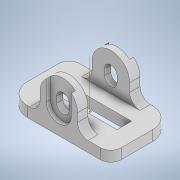
# Autodesk Inventor part: 15-1
Saved by Autodesk Inventor 2022 (Build 260153000, 153)
## iProperties
Created: 2021-09-25
Part Number: 15-1
Material: 일반
Document SubType Name: Modeling
Designer: 서울공업고등학교
Density: 1 g/cm^3
Appearance: 기본값
Author: 서울공업고등학교
Autodesk Inventor part; units mm, degrees
ref_plane "YZ Plane" through (0, 0, 0) normal (1, 0, 0) x (0, 1, 0)
ref_plane "XZ Plane" through (0, 0, 0) normal (0, 1, 0) x (-1, 0, 0)
ref_plane "XY Plane" through (0, 0, 0) normal (0, 0, 1) x (1, 0, 0)
sketch "스케치1" plane through (0, 0, 0) normal (0, 0, 1) x (1, 0, 0)
  line L0 (-25, 2.5) -> (-25, -2.5)
  line L1 (25, -2.5) -> (25, 2.5)
  line L2 (-25, -2.5) -> (25, -2.5)
  arc A0 (9, 11.5) -> (-9, 11.5) centre (0, 11.5) ccw
  line L3 (0, 11.5) -> (0, 8.5) construction
  line L4 (-3, 11.5) -> (-3, 8.5)
  line L5 (3, 8.5) -> (3, 11.5)
  arc A1 (3, 11.5) -> (-3, 11.5) centre (0, 11.5) ccw
  arc A2 (-3, 8.5) -> (3, 8.5) centre (0, 8.5) ccw
  line L6 (0, 20.1537) -> (0, 8.5) construction
  line L7 (-6, 18.2082) -> (-6, 8.5)
  line L8 (6, 8.5) -> (6, 18.2082)
  arc A3 (-6, 8.5) -> (6, 8.5) centre (0, 8.5) ccw
  line L9 (0, -7.1) -> (0, 25.1) projected
  line L10 (-9, 11.5) -> (-9, 2.5)
  line L11 (9, 11.5) -> (9, 2.5)
  line L12 (25, 2.5) -> (9, 2.5)
  line L13 (-9, 2.5) -> (-25, 2.5)
  point P0 (-25, 0)
  point P1 (0, 0)
  point P2 (0, 10)
  point P3 (0, 14.3269)
  dimension "d7" = 50
  dimension "d8" = 5
  dimension "d9" = 25
  dimension "d10" = 18
  dimension "d11" = 3
  dimension "d14" = 0
  dimension "d15" = 0
  constraints: 30 end point, 12 tangent, 10 point on circle, 6 perpendicular, 4 centre point, 3 horizontal, 3 midpoint, 3 parallel, 2 vertical, 1 horizontal alignment
  measures "d7" distance of L1.end L0.start
  measures "d8" distance of L0.start L0.end
  measures "d9" distance from line of point (0, 0) L0
  measures "d10" diameter of A0
  measures "d11" distance of L3.start L3.end
  measures "d14" distance from line of L9 point (0, 14.327)
  measures "d15" horizontal distance of point (0, 14.327) point (0, 10)
extrude "돌출1" add sketch "스케치1" along normal mid plane 30 contours L13 L10 A0 L7 A3 L9 L2 L0 | L9 A3 L8 A0 L11 L12 L1 L2
extrude "돌출2" add sketch "스케치1" along normal mid plane 26 contours L9 A2 L5 A1 A0 L8 A3 | A3 L7 A0 L9 A1 L4 A2
fillet "모깎기1" radius 5 2 edges at (9, 2.5, 0) (-9, 2.5, 0)
sketch "스케치3" plane through (0, 0, 0) normal (0, 0, 1) x (1, 0, 0)
  line L0 (-23.0758, 32.485) -> (23.2904, 32.485)
  line L1 (23.2904, 32.485) -> (23.2904, 2.5)
  line L2 (23.2904, 2.5) -> (-23.0758, 2.5)
  line L3 (-23.0758, 2.5) -> (-23.0758, 32.485)
  line L4 (-25, 2.5) -> (-14, 2.5) projected
  point P0 (0, 0)
  dimension "d21" = 0
  constraints: 8 end point, 2 parallel, 1 horizontal, 1 perpendicular
  measures "d21" distance between parallel lines of L2 L4
extrude "돌출3" cut sketch "스케치3" along normal mid plane 20
sketch "스케치4" plane through (-25, 2.5, 15) normal (0, 1, 0) x (1, 0, 0)
  line L0 (8.5, 18.5) -> (41.5, 18.5)
  line L1 (41.5, 18.5) -> (41.5, 11.5)
  line L2 (41.5, 11.5) -> (8.5, 11.5)
  line L3 (8.5, 11.5) -> (8.5, 18.5)
  line L4 (8.5, 18.5) -> (41.5, 11.5) construction
  line L5 (41.5, 18.5) -> (8.5, 11.5) construction
  point P0 (25, 15)
  dimension "d24" = 33
  dimension "d25" = 7
  constraints: 12 end point, 2 midpoint, 2 parallel, 1 horizontal, 1 perpendicular
  measures "d24" distance of L1.end L2.end
  measures "d25" distance of L0.end L1.end
extrude "돌출4" cut sketch "스케치4" against normal blind 20
fillet "모깎기2" radius 5 2 edges at (-25, 0, -15) (25, 0, 15)
fillet "모깎기3" radius 10 2 edges at (-25, 0, 15) (25, 0, -15)
